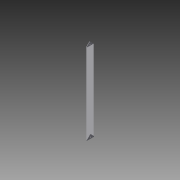
# Autodesk Inventor part: cross brace
Saved by Autodesk Inventor 2015 SP1 (Build 190203100, 203)
## iProperties
Created: 2015-01-19
Part Number: cross brace
Material: Generic
Document SubType Name: Modeling
Designer: Jarod
Density: 1 g/cm^3
Appearance: Default
Author: Jarod
Autodesk Inventor part; units mm, degrees
ref_plane "YZ Plane" through (0, 0, 0) normal (1, 0, 0) x (0, 1, 0)
ref_plane "XZ Plane" through (0, 0, 0) normal (0, 1, 0) x (-1, 0, 0)
ref_plane "XY Plane" through (0, 0, 0) normal (0, 0, 1) x (1, 0, 0)
sketch "Sketch1" plane through (0, 0, 0) normal (0, 1, 0) x (-1, 0, 0)
  line L0 (0, 0) -> (527.05, 0) construction
  line L1 (527.05, 0) -> (527.05, 787.4) construction
  line L2 (527.05, 787.4) -> (0, 787.4) construction
  line L3 (0, 787.4) -> (0, 0) construction
  line L4 (0, 787.4) -> (527.05, 0)
  line L5 (527.05, 0) -> (527.05, 50.8)
  line L6 (527.05, 0) -> (577.85, 0) construction
  line L7 (0, 787.4) -> (0, 838.2)
  line L8 (0, 787.4) -> (50.8, 787.4) construction
  line L9 (0, 838.2) -> (527.05, 50.8)
  dimension "d0" = 527.05
  dimension "d1" = 787.4
  dimension "d2" = 50.8
  dimension "d3" = 90
  dimension "d4" = 50.8
  dimension "d5" = 90
  constraints: 20 end point, 3 horizontal, 3 perpendicular, 2 parallel, 1 collinear, 1 vertical
  measures "d0" distance of L2.end L1.end
  measures "d1" distance of L1.end L0.end
  measures "d2" distance of L0.end L5.end
  measures "d3" angle of L6 L5
  measures "d4" distance of L2.end L7.end
  measures "d5" angle of L8 L7
extrude "Extrusion1" add sketch "Sketch1" along normal blind 3.175
sketch "Sketch6" plane through (-527.05, 0, 0) normal (-1, 0, 0) x (0, 0, 1)
  line L0 (50.8, 0) -> (0, 0) projected
  line L1 (50.8, 0) -> (50.8, 3.175) projected
  line L2 (0, 3.175) -> (50.8, 3.175) projected
  line L3 (0, 0) -> (0, 3.175) projected
  line L4 (50.8, 0) -> (25.4, -25.4)
  line L5 (50.8, 0) -> (86.721, 0) construction
  line L6 (25.4, -25.4) -> (0, 0)
  dimension "d33" = 135
  constraints: 6 end point, 1 equal length, 1 horizontal, 1 perpendicular
  measures "d33" angle of L4 L5
extrude "Extrusion4" add sketch "Sketch6" against normal blind 3.175
sketch "Sketch8" plane through (0, 3.175, 0) normal (0, 1, 0) x (1, 0, 0)
  line L0 (-527.05, 0) -> (-527.05, -50.8) projected
  line L1 (-527.05, -50.8) -> (0, -838.2) projected
  line L2 (0, -838.2) -> (0, -787.4) projected
  line L3 (0, -787.4) -> (-523.875, -4.7434) projected
  line L4 (-523.875, 0) -> (-523.875, -4.7434) projected
  line L5 (-527.05, 0) -> (-523.875, 0) projected
  line L6 (0, -838.2) -> (0, -812.8)
  line L7 (0, -787.4) -> (0, -838.2) projected
  line L8 (0, -812.8) -> (-17.0016, -812.8)
  line L9 (-17.0016, -812.8) -> (0, -838.2)
  line L10 (0, -838.2) -> (-527.05, -50.8) projected
  point P0 (0, 0)
  constraints: 6 end point, 1 collinear, 1 midpoint, 1 perpendicular, 1 point on line
extrude "Extrusion6" cut sketch "Sketch8" against normal blind 3.175 contours L8 L2 L1
body "Solid1"
